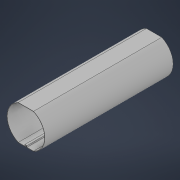
# Autodesk Inventor part: PodShell
Saved by Autodesk Inventor 2021 (Build 250183000, 183)
## iProperties
Created: 2021-01-31
Part Number: PodShell
Material: Generic
Document SubType Name: Modeling
Designer: argon
Density: 1 g/cm^3
Appearance: Light Gray
Author: argon
Autodesk Inventor part; units mm, degrees
ref_plane "YZ Plane" through (0, 0, 0) normal (1, 0, 0) x (0, 1, 0)
ref_plane "XZ Plane" through (0, 0, 0) normal (0, 1, 0) x (-1, 0, 0)
ref_plane "XY Plane" through (0, 0, 0) normal (0, 0, 1) x (1, 0, 0)
sketch "Sketch1" plane through (0, 0, 0) normal (0, 0, 1) x (1, 0, 0)
  circle A0 centre (0, 0) radius 1783
  circle A1 centre (0, 0) radius 1750
  line L0 (-786.8221, -1600) -> (786.8221, -1600)
  line L1 (-786.8221, 1600) -> (786.8221, 1600)
  line L2 (-715.8212, 1633) -> (715.8212, 1633)
  line L3 (-715.8212, -1633) -> (715.8212, -1633)
  line L4 (-64, -1498) -> (64, -1498)
  line L5 (64, -1498) -> (64, -1600)
  line L6 (64, -1600) -> (-64, -1600)
  line L7 (-64, -1600) -> (-64, -1498)
  line L8 (-64, -1498) -> (64, -1600) construction
  line L9 (64, -1498) -> (-64, -1600) construction
  line L10 (-97, -1633) -> (97, -1633)
  line L11 (97, -1633) -> (97, -1465)
  line L12 (97, -1465) -> (-97, -1465)
  line L13 (-97, -1465) -> (-97, -1633)
  line L14 (-97, -1633) -> (97, -1465) construction
  line L15 (97, -1633) -> (-97, -1465) construction
  line L16 (-64, -1600) -> (-64, -1633)
  line L17 (64, -1600) -> (64, -1633)
  point P0 (0, -1549)
  point P1 (0, -1549)
  point P2 (97, -1600)
  point P3 (-97, -1600)
  point P4 (-708.8723, -1600)
  point P5 (-708.8723, 1600)
  point P6 (708.8723, 1600)
  point P7 (708.8723, -1600)
  point P8 (97, -1633)
  dimension "d0" = 3566
  dimension "d1" = 33
  dimension "d2" = 1600
  dimension "d3" = 1600
  dimension "d4" = 33
  dimension "d5" = 33
  dimension "d6" = 33
  dimension "d7" = 33
  dimension "d8" = 102
  dimension "d9" = 128
  constraints: 36 end point, 6 parallel, 5 midpoint, 4 horizontal, 3 perpendicular, 3 point on line, 2 coincident, 1 centre point, 1 vertical, 1 vertical alignment, 10 other
  measures "d2" distance from line of L0 point (0, 0)
  measures "d3" distance from line of point (0, 0) L1
  measures "d4" distance between parallel lines of L3 L0
  measures "d5" distance between parallel lines of L1 L2
  measures "d6" distance between parallel lines of L5 L11
  measures "d7" distance between parallel lines of L4 L12
  measures "d8" distance of L4.end L5.end
  measures "d9" distance of L4.start L4.end
extrude "Extrusion1" add sketch "Sketch1" along normal blind 12000 contours A0 L0 A1 L1 | L1 A1 L2 A0 | A0 L3 A1 L0 | L1 A1 L2 | A1 L3 L11 L0 | L2 A1 L1 A0 | A1 L0 A0 L1 | A0 L0 A1 L3 | L11 L3 L17 L0 | L0 L5 L4 L7 L13 L12 L11 | L0 L13 L3 A1 | L0 L16 L3 L13
body "Solid1"
